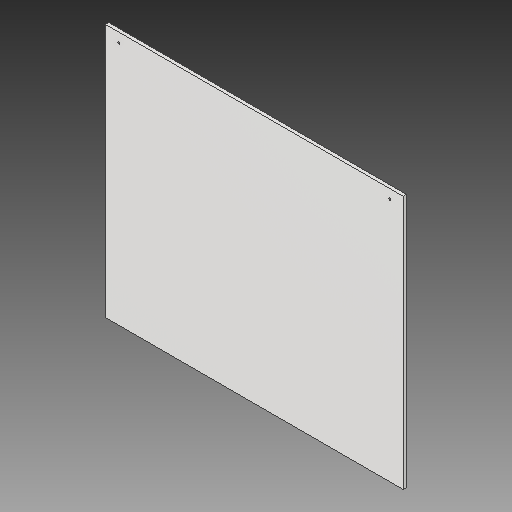
# Autodesk Inventor part: 56.25x48 Gyp Top
Saved by Autodesk Inventor 2017 (Build 210142000, 142)
## iProperties
Created: 2017-05-26
Part Number: 56.25x48 Gyp Top
Material: Generic
Document SubType Name: Modeling
Designer: cas7
Density: 1 g/cm^3
Appearance: Default
Mass: 27650.4 g
Surface Area: 35686.4 cm^2
Volume: 27650.4 cm^3
Author: cas7
Autodesk Inventor part; units mm, degrees
ref_plane "YZ Plane" through (0, 0, 0) normal (1, 0, 0) x (0, 1, 0)
ref_plane "XZ Plane" through (0, 0, 0) normal (0, 1, 0) x (-1, 0, 0)
ref_plane "XY Plane" through (0, 0, 0) normal (0, 0, 1) x (1, 0, 0)
sketch "Sketch1" plane through (0, 0, 0) normal (0, 0, 1) x (1, 0, 0)
  line L0 (0, 0) -> (1428.75, 0)
  line L1 (1428.75, 0) -> (1428.75, 1219.2)
  line L2 (1428.75, 1219.2) -> (0, 1219.2)
  line L3 (0, 1219.2) -> (0, 0)
  dimension "d0" = 1428.75
  dimension "d1" = 1219.2
  constraints: 8 end point, 2 parallel, 1 horizontal, 1 perpendicular
  measures "d0" distance of L2.end L1.end
  measures "d1" distance of L1.end L0.end
extrude "Extrusion1" add sketch "Sketch1" along normal blind 15.875
sketch "Sketch2" plane through (0, 0, 15.875) normal (0, 0, 1) x (1, 0, 0)
  line L0 (1428.75, 1219.2) -> (1365.25, 1219.2)
  line L1 (1365.25, 1219.2) -> (1365.25, 1174.75)
  line L2 (1365.25, 1174.75) -> (1428.75, 1174.75)
  line L3 (1428.75, 1174.75) -> (1428.75, 1219.2)
  line L4 (0, 1219.2) -> (63.5, 1219.2)
  line L5 (63.5, 1219.2) -> (63.5, 1174.75)
  line L6 (63.5, 1174.75) -> (0, 1174.75)
  line L7 (0, 1174.75) -> (0, 1219.2)
  dimension "d4" = 63.5
  dimension "d5" = 44.45
  dimension "d6" = 63.5
  constraints: 16 end point, 4 parallel, 2 coincident, 2 horizontal, 2 perpendicular, 1 point on line
  measures "d4" distance of L2.end L1.end
  measures "d5" distance of L1.end L0.end
  measures "d6" distance of L5.end L6.end
hole "Hole1" at (1365.25, 1174.75, 15.875) at (63.5, 1174.75, 15.875) direction (0, 0, -1) diameter 10.5918 depth 35.179 tip angle 118 thread size "1/2-13 UNC" class "2B" standard "ANSI Unified Screw Threads"
body "Solid1"
